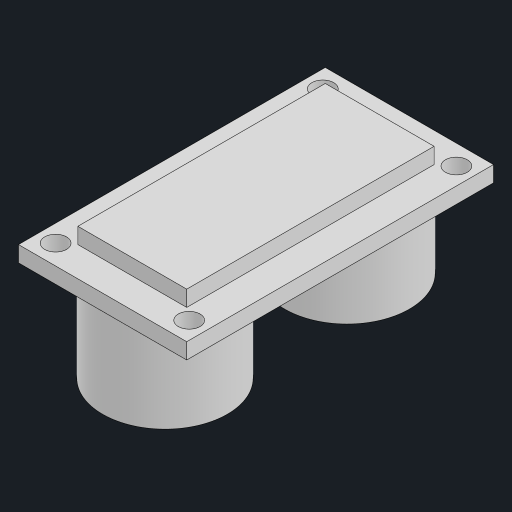
# Autodesk Inventor part: UltrasonicSensor
Saved by Autodesk Inventor 2023 (Build 270158000, 158)
## iProperties
Created: 2022-06-24
Part Number: UltrasonicSensor
Material: 一般
Document SubType Name: Modeling
Designer: legot
Density: 1 g/cm^3
Appearance: 既定
Author: legot
Autodesk Inventor part; units mm, degrees
ref_plane "YZ Plane" through (0, 0, 0) normal (1, 0, 0) x (0, 1, 0)
ref_plane "XZ Plane" through (0, 0, 0) normal (0, 1, 0) x (-1, 0, 0)
ref_plane "XY Plane" through (0, 0, 0) normal (0, 0, 1) x (1, 0, 0)
sketch "スケッチ1" plane through (0, 0, 0) normal (0, 1, 0) x (-1, 0, 0)
  line L0 (8.5, 15.5) -> (-8.5, 15.5)
  line L1 (-8.5, 15.5) -> (-8.5, -15.5)
  line L2 (-8.5, -15.5) -> (8.5, -15.5)
  line L3 (8.5, -15.5) -> (8.5, 15.5)
  circle A0 centre (0, 9.2) radius 6.3
  circle A1 centre (0, -9.2) radius 6.3
  circle A2 centre (6.75, -13.5) radius 1.1
  line L4 (6.75, -13.5) -> (-6.75, -13.5) construction
  line L5 (-6.75, -13.5) -> (-6.75, 13.5) construction
  line L6 (-6.75, 13.5) -> (6.75, 13.5) construction
  line L7 (6.75, 13.5) -> (6.75, -13.5) construction
  circle A3 centre (-6.75, -13.5) radius 1.1
  circle A4 centre (6.75, 13.5) radius 1.1
  circle A5 centre (-6.75, 13.5) radius 1.1
  point P0 (0, 0)
  point P1 (0, 15.5)
  point P2 (8.5, 0)
  point P3 (6.75, 0)
  point P4 (0, 13.5)
  dimension "d0" = 17
  dimension "d1" = 31
  dimension "d2" = 12.6
  dimension "d10" = 2.2
  dimension "d11" = 27
  dimension "d12" = 13.5
  dimension "d13" = 2.2
  dimension "d14" = 2.2
  dimension "d15" = 2.2
  dimension "d16" = 9.2
  constraints: 16 end point, 6 centre point, 4 coincident, 4 midpoint, 4 parallel, 4 vertical alignment, 2 horizontal, 2 horizontal alignment, 2 perpendicular, 2 tangent, 1 equal radius
  measures "d0" distance of L0.start L0.end
  measures "d1" distance of L2.end L0.start
  measures "d2" diameter of A0
  measures "d10" diameter of A2
  measures "d11" distance of L6.end L4.start
  measures "d12" distance of L4.start L4.end
  measures "d13" diameter of A3
  measures "d14" diameter of A4
  measures "d15" diameter of A5
  measures "d16" distance of A0.centre point (0, 0)
extrude "押し出し1" add sketch "スケッチ1" along normal blind 1.6 contours A0 | A1 | L3 L2 L1 L0
extrude "押し出し2" add sketch "スケッチ1" against normal blind 9 contours A0 | A1
sketch "スケッチ2" plane through (0, 1.6, 0) normal (0, 1, 0) x (1, 0, 0)
  line L0 (8.5, 15.5) -> (-8.5, 15.5) projected
  line L1 (-8.5, 15.5) -> (-8.5, -15.5) projected
  line L2 (-8.5, -15.5) -> (8.5, -15.5) projected
  line L3 (8.5, -15.5) -> (8.5, 15.5) projected
  line L4 (-5.5, -12.5) -> (-5.5, 12.5)
  line L5 (-5.5, 12.5) -> (5.5, 12.5)
  line L6 (5.5, 12.5) -> (5.5, -12.5)
  line L7 (5.5, -12.5) -> (-5.5, -12.5)
  point P0 (0, 0)
  dimension "d7" = 3
  constraints: 8 end point, 3 other
  measures "d7" distance between parallel lines of L1 L4
extrude "押し出し3" add sketch "スケッチ2" along normal blind 1.6 contours L4 L5 L6 L7
